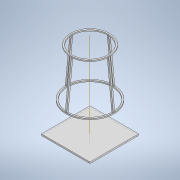
# Autodesk Inventor part: Hub
Saved by Autodesk Inventor 2022 (Build 260153000, 153)
## iProperties
Created: 2022-01-10
Part Number: Hub
Material: Generic
Document SubType Name: Modeling
Designer: Daniel Marquez
Density: 1 g/cm^3
Appearance: Default
Author: Daniel Marquez
Autodesk Inventor part; units mm, degrees
ref_plane "YZ Plane" through (0, 0, 0) normal (1, 0, 0) x (0, 1, 0)
ref_plane "XY Plane" through (0, 0, 0) normal (0, 0, 1) x (1, 0, 0)
ref_plane "Work Plane1" through (0, 2641.6, 0) normal (0, 1, 0) x (-1, 0, 0)
sketch "Sketch1" plane through (0, 2641.6, 0) normal (0, 1, 0) x (-1, 0, 0)
  circle A0 centre (0, 0) radius 609.6
  circle A1 centre (0, 0) radius 660.4
  line L0 (0, 660.4) -> (0, 609.6)
  line L1 (-609.6, 0) -> (-660.4, 0)
  dimension "d1" = 1219.2
  dimension "d2" = 1320.8
  constraints: 4 end point, 4 point on circle, 2 centre point, 2 coincident, 1 perpendicular, 1 vertical
  measures "d1" diameter of A0
  measures "d2" diameter of A1
extrude "Extrusion1" add sketch "Sketch1" along normal blind 38.1 contours A0 L0 A1 L1 | A0 L1 A1 L0
ref_plane "Work Plane2" through (0, 1041.4, 0) normal (0, 1, 0) x (-1, 0, 0)
sketch "Sketch2" plane through (0, 1041.4, 0) normal (0, 1, 0) x (-1, 0, 0)
  circle A0 centre (0, 0) radius 763.5875
  circle A1 centre (0, 0) radius 814.3875
  line L0 (0, 763.5875) -> (0, 814.3875)
  dimension "d6" = 1527.175
  dimension "d7" = 1628.775
  constraints: 2 coincident, 2 end point, 2 vertical alignment, 1 vertical, 4 other
extrude "Extrusion2" add sketch "Sketch2" along normal blind 38.1
sketch "Sketch3" plane through (0, 0, 0) normal (0, 0, 1) x (1, 0, 0)
  line L0 (814.3875, 1079.5) -> (-814.3875, 1079.5) projected
  line L1 (763.5875, 1079.5) -> (814.3875, 1079.5)
  line L2 (660.4, 2641.6) -> (-660.4, 2641.6) projected
  line L3 (609.6, 2641.6) -> (660.4, 2641.6)
  line L4 (660.4, 2641.6) -> (814.3875, 1079.5)
  line L5 (763.5875, 1079.5) -> (609.6, 2641.6)
  point P0 (0, 0)
  constraints: 8 end point, 2 collinear, 2 point on line, 1 parallel
extrude "Extrusion3" add sketch "Sketch3" along normal mid plane 50.8
pattern_circular "Circular Pattern1" count 4 over 360 about axis through (0, -10, 0) along (0, 1, 0) of "Extrusion3"
sketch "Sketch4" plane through (0, 0, 0) normal (0, 1, 0) x (-1, 0, 0)
  line L0 (825.5, -825.5) -> (-825.5, -825.5)
  line L1 (-825.5, -825.5) -> (-825.5, 825.5)
  line L2 (-825.5, 825.5) -> (825.5, 825.5)
  line L3 (825.5, 825.5) -> (825.5, -825.5)
  line L4 (825.5, -825.5) -> (-825.5, 825.5) construction
  line L5 (-825.5, -825.5) -> (825.5, 825.5) construction
  point P0 (0, 0)
  dimension "d15" = 1651
  dimension "d16" = 1651
  constraints: 12 end point, 2 midpoint, 2 parallel, 1 horizontal, 1 perpendicular
  measures "d15" distance of L1.end L2.end
  measures "d16" distance of L0.end L1.end
extrude "Extrusion4" add sketch "Sketch4" along normal blind 50.8
body "Solid1"
